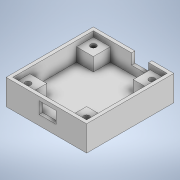
# Autodesk Inventor part: PCB_REMOTE_Holder_tall_
Saved by Autodesk Inventor 2021 (Build 250183000, 183)
## iProperties
Created: 2021-04-21
Part Number: PCB_REMOTE_Holder_tall_
Material: Generic
Document SubType Name: Modeling
Designer: Patrick
Density: 1 g/cm^3
Appearance: Default
Author: Patrick
Autodesk Inventor part; units mm, degrees
ref_plane "YZ Plane" through (0, 0, 0) normal (1, 0, 0) x (0, 1, 0)
ref_plane "XZ Plane" through (0, 0, 0) normal (0, 1, 0) x (-1, 0, 0)
ref_plane "XY Plane" through (0, 0, 0) normal (0, 0, 1) x (1, 0, 0)
sketch "Sketch1" plane through (0, 0, 0) normal (0, 1, 0) x (-1, 0, 0)
  line L0 (0, 0) -> (47.635, 0)
  line L1 (47.635, 0) -> (47.635, -52.715)
  line L2 (47.635, -52.715) -> (0, -52.715)
  line L3 (0, -52.715) -> (0, 0)
  circle A0 centre (45.725, -1.91) radius 2.1
  circle A1 centre (45.725, -50.805) radius 2.1
  circle A2 centre (1.91, -1.91) radius 2.1
  circle A3 centre (1.91, -50.805) radius 2.1
  line L4 (47.635, 0) -> (51.445, 0)
  line L5 (51.445, 0) -> (51.445, -52.715)
  line L6 (51.445, -52.715) -> (47.635, -52.715)
  line L7 (47.635, -52.715) -> (47.635, 0)
  line L8 (0, 0) -> (-3.81, 0)
  line L9 (-3.81, 0) -> (-3.81, -56.525)
  line L10 (-3.81, -56.525) -> (0, -56.525)
  line L11 (0, -56.525) -> (0, 0)
  line L12 (51.445, -52.715) -> (-6.35, -52.715)
  line L13 (-6.35, -52.715) -> (-6.35, -56.525)
  line L14 (-6.35, -56.525) -> (51.445, -56.525)
  line L15 (51.445, -56.525) -> (51.445, -52.715)
  line L16 (-3.81, 0) -> (51.445, 0)
  line L17 (51.445, 0) -> (51.445, 3.81)
  line L18 (51.445, 3.81) -> (-3.81, 3.81)
  line L19 (-3.81, 3.81) -> (-3.81, 0)
  point P0 (0, -52.715)
  point P1 (0, -51.6779)
  point P2 (0, -49.9321)
  point P3 (0, -2.7829)
  point P4 (0, -1.0371)
  point P5 (-3.81, -77.675)
  point P6 (-3.81, -52.715)
  point P7 (0, -52.715)
  point P8 (1.0371, -52.715)
  point P9 (2.7829, -52.715)
  point P10 (0, -52.715)
  point P11 (0, -56.525)
  point P12 (0, -56.525)
  dimension "d0" = 52.715
  dimension "d1" = 47.635
  dimension "d3" = 4.2
  dimension "d4" = 4.2
  dimension "d6" = 1.91
  dimension "d7" = 1.91
  dimension "d8" = 1.91
  dimension "d9" = 4.2
  dimension "d10" = 4.2
  dimension "d11" = 1.91
  dimension "d12" = 1.91
  dimension "d13" = 1.91
  dimension "d14" = 1.91
  dimension "d15" = 1.91
  dimension "d18" = 3.81
  dimension "d19" = 3.81
  dimension "d20" = 3.81
  dimension "d21" = 3.81
  dimension "d38" = 0
  dimension "d39" = 0
  constraints: 40 end point, 10 parallel, 5 horizontal, 5 perpendicular, 4 centre point, 1 point on line
  measures "d0" distance of L2.end L0.start
  measures "d1" distance between parallel lines of L3 L1
  measures "d3" diameter of A1
  measures "d4" diameter of A0
  measures "d6" distance from line of L1 A0.centre
  measures "d7" distance from line of L2 A1.centre
  measures "d8" distance from line of A0.centre L0
  measures "d9" diameter of A2
  measures "d10" diameter of A3
  measures "d11" distance from line of L0 A2.centre
  measures "d12" distance from line of A2.centre L3
  measures "d13" distance from line of L2 A3.centre
  measures "d14" distance from line of L3 A3.centre
  measures "d15" distance from line of L1 A1.centre
  measures "d18" distance of L5.end L6.end
  measures "d19" distance of L10.end L9.end
  measures "d20" distance of L13.end L12.end
  measures "d21" distance of L17.end L16.end
  measures "d38" distance between parallel lines of L2 L12
  measures "d39" distance between parallel lines of L14 L10
extrude "Extrusion5" add sketch "Sketch1" along normal blind 15 contours L8 L19 L18 L17 L4 L0 A0 A2 | L0 A2 L3 | L3 A2 A3 L12 L9 L8 | L0 A0 L1 A1 L2 A3 L3 A2 | L12 L11 L10 L9 | L3 A3 L2 | L2 A3 A1 L6 L15 L14 L11 | L0 L1 A0 | A0 L1 L4 L5 L6 A1 | L1 L2 A1 picked at (0.2904, -0.2904) picked at (0.2904, -52.4246) picked at (47.3446, -0.2904) picked at (47.3446, -52.4246)
sketch "Sketch6" plane through (0, 15, 0) normal (0, 1, 0) x (1, 0, 0)
  line L0 (-51.445, -3.81) -> (3.81, -3.81) projected
  line L1 (-51.445, -3.81) -> (-38.745, -3.81)
  line L2 (-38.745, -3.81) -> (-38.745, 8.89)
  line L3 (-38.745, 8.89) -> (-51.445, 8.89)
  line L4 (-51.445, 8.89) -> (-51.445, -3.81)
  line L5 (3.81, 56.525) -> (-51.445, 56.525) projected
  line L6 (-51.445, 56.525) -> (-38.745, 56.525)
  line L7 (-38.745, 56.525) -> (-38.745, 43.825)
  line L8 (-38.745, 43.825) -> (-51.445, 43.825)
  line L9 (-51.445, 43.825) -> (-51.445, 56.525)
  line L10 (3.81, -3.81) -> (3.81, 56.525) projected
  line L11 (3.81, 56.525) -> (-8.89, 56.525)
  line L12 (-8.89, 56.525) -> (-8.89, 43.825)
  line L13 (-8.89, 43.825) -> (3.81, 43.825)
  line L14 (3.81, 43.825) -> (3.81, 56.525)
  line L15 (3.81, -3.81) -> (-8.89, -3.81)
  line L16 (-8.89, -3.81) -> (-8.89, 8.89)
  line L17 (-8.89, 8.89) -> (3.81, 8.89)
  line L18 (3.81, 8.89) -> (3.81, -3.81)
  line L19 (3.81, 56.525) -> (-51.445, 56.525) projected
  line L20 (-51.445, 56.525) -> (-51.445, -3.81) projected
  line L21 (-51.445, -3.81) -> (3.81, -3.81) projected
  line L22 (3.81, -3.81) -> (3.81, 56.525) projected
  circle A0 centre (-1.91, 1.91) radius 2.1 projected
  circle A1 centre (-45.725, 1.91) radius 2.1 projected
  circle A2 centre (-45.725, 50.805) radius 2.1 projected
  circle A3 centre (-1.91, 50.805) radius 2.1 projected
  point P0 (0, 0)
  point P1 (3.81, 8.89)
  dimension "d42" = 12.7
  dimension "d43" = 12.7
  dimension "d44" = 12.7
  dimension "d45" = 12.7
  dimension "d46" = 12.7
  dimension "d47" = 12.7
  constraints: 32 end point, 8 parallel, 4 horizontal, 4 perpendicular
  measures "d42" distance of L3.end L2.end
  measures "d43" distance of L2.end L1.end
  measures "d44" distance of L7.end L8.end
  measures "d45" distance of L6.end L7.end
  measures "d46" distance of L13.end L12.end
  measures "d47" distance of L12.end L11.end
extrude "Extrusion6" cut sketch "Sketch6" against normal blind 10 contours L2 L3 L20 L8 L7 L5 L12 L13 L10 L17 L16 L0
sketch "Sketch7" plane through (0, 0, 0) normal (0, -1, 0) x (1, 0, 0)
  line L0 (3.81, -56.525) -> (-51.445, -56.525) projected
  line L1 (3.81, 3.81) -> (3.81, -56.525) projected
  line L2 (-51.445, 3.81) -> (3.81, 3.81) projected
  line L3 (-51.445, -56.525) -> (-51.445, 3.81) projected
  circle A0 centre (-1.91, -1.91) radius 2.1 projected
  circle A1 centre (-45.725, -1.91) radius 2.1 projected
  circle A2 centre (-45.725, -50.805) radius 2.1 projected
  circle A3 centre (-1.91, -50.805) radius 2.1 projected
  line L4 (-8.89, 3.81) -> (3.81, 3.81) projected
  line L5 (3.81, 3.81) -> (-51.445, 3.81)
  line L6 (-51.445, 3.81) -> (-51.445, 6.35)
  line L7 (-51.445, 6.35) -> (3.81, 6.35)
  line L8 (3.81, 6.35) -> (3.81, 3.81)
  line L9 (-51.445, 6.35) -> (-53.985, 6.35)
  line L10 (-53.985, 6.35) -> (-53.985, -56.525)
  line L11 (-53.985, -56.525) -> (-51.445, -56.525)
  line L12 (-51.445, -56.525) -> (-51.445, 6.35)
  line L13 (-53.985, -56.525) -> (3.81, -56.525)
  line L14 (3.81, -56.525) -> (3.81, -59.065)
  line L15 (3.81, -59.065) -> (-53.985, -59.065)
  line L16 (-53.985, -59.065) -> (-53.985, -56.525)
  line L17 (3.81, -59.065) -> (6.35, -59.065)
  line L18 (6.35, -59.065) -> (6.35, 5.08)
  line L19 (6.35, 5.08) -> (3.81, 5.08)
  line L20 (3.81, 5.08) -> (3.81, -59.065)
  line L21 (6.35, 5.08) -> (3.81, 5.08)
  line L22 (3.81, 5.08) -> (3.81, 6.35)
  line L23 (3.81, 6.35) -> (6.35, 6.35)
  line L24 (6.35, 6.35) -> (6.35, 5.08)
  point P0 (0, 0)
  dimension "d50" = 2.54
  dimension "d51" = 2.54
  dimension "d52" = 2.54
  dimension "d53" = 2.54
  constraints: 40 end point, 10 parallel, 5 horizontal, 5 perpendicular, 1 point on line
  measures "d50" distance of L5.end L6.end
  measures "d51" distance of L11.end L10.end
  measures "d52" distance of L13.end L14.end
  measures "d53" distance of L19.end L18.end
extrude "Extrusion7" add sketch "Sketch7" against normal blind 19 contours L14 L15 L16 L11 L0 | L1 L8 L19 L18 L17 L14 | L11 L10 L9 L6 L3 | L2 L6 L7 L8 | L8 L23 L24 L19
sketch "Sketch8" plane through (0, 19, 0) normal (0, 1, 0) x (1, 0, 0)
  line L0 (-53.985, -6.35) -> (6.35, -6.35) projected
  line L1 (6.35, -6.35) -> (6.35, 59.065) projected
  line L2 (6.35, 59.065) -> (-53.985, 59.065) projected
  line L3 (-53.985, 59.065) -> (-53.985, -6.35) projected
  line L4 (3.81, 56.525) -> (3.81, -3.81) projected
  line L5 (3.81, -3.81) -> (-51.445, -3.81) projected
  line L6 (-51.445, -3.81) -> (-51.445, 56.525) projected
  line L7 (-51.445, 56.525) -> (3.81, 56.525) projected
  circle A0 centre (-1.91, 50.805) radius 2.1 projected
  line L8 (-1.91, 50.805) -> (-10.17, 50.805)
  line L9 (-10.17, 50.805) -> (-10.17, 48.127)
  line L10 (-10.17, 48.127) -> (-1.91, 48.127)
  line L11 (-1.91, 48.127) -> (-1.91, 50.805)
  line L12 (6.35, 59.065) -> (-53.985, 59.065) projected
  line L13 (-10.17, 48.127) -> (-22.87, 48.127)
  line L14 (-22.87, 48.127) -> (-22.87, 59.065)
  line L15 (-22.87, 59.065) -> (-10.17, 59.065)
  line L16 (-10.17, 59.065) -> (-10.17, 48.127)
  point P0 (0, 0)
  point P1 (-10.17, 56.525)
  point P2 (-22.87, 56.525)
  dimension "d56" = 8.26
  dimension "d57" = 12.7
  constraints: 16 end point, 4 parallel, 2 horizontal, 2 perpendicular, 1 point on line
  measures "d56" distance of L10.end L9.end
  measures "d57" distance of L14.end L15.end
extrude "Extrusion8" cut sketch "Sketch8" against normal blind 8 contours L2 L16 L7 L14
sketch "Sketch9" plane through (0, 5, 0) normal (0, 1, 0) x (1, 0, 0)
  point P0 (0, 0)
sketch "Sketch10" plane through (3.81, 19, 3.81) normal (0, 0, -1) x (-1, 0, 0)
  line L0 (33.02, -2.8033) -> (20.32, -2.8033)
  line L1 (20.32, -2.8033) -> (20.32, -11.7199)
  line L2 (20.32, -11.7199) -> (33.02, -11.7199)
  line L3 (33.02, -11.7199) -> (33.02, -2.8033)
  point P0 (3.81, -19)
  point P1 (12.7, -4)
  dimension "d60" = 12.7
  dimension "d61" = 7.62
  constraints: 8 end point, 2 parallel, 1 horizontal, 1 perpendicular
  measures "d60" distance of L2.end L1.end
  measures "d61" distance from line of L1 point (12.7, -4)
extrude "Extrusion9" cut sketch "Sketch10" against normal blind 25.4
body "Solid3"
